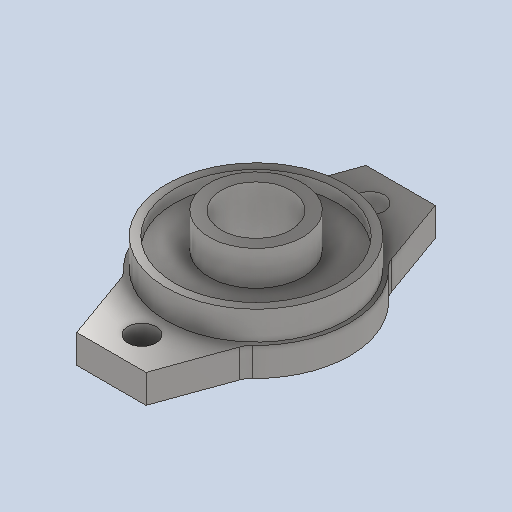
# Autodesk Inventor part: HCMUTE-CDT23-GOI_DO_PHI-17
Saved by Autodesk Inventor 2023 (Build 270158000, 158)
## iProperties
Created: 2023-11-19
Part Number: HCMUTE-CDT23-GOI_DO_PHI-17
Material: Stainless Steel
Document SubType Name: Modeling
Designer: havie
Mass: 171.361 g
Surface Area: 85.9405 cm^2
Volume: 21.4202 cm^3
Density: 8 g/cm^3
Appearance: Semi-Polished
Author: havie
Autodesk Inventor part; units mm, degrees
ref_plane "YZ Plane" through (0, 0, 0) normal (1, 0, 0) x (0, 1, 0)
ref_plane "XZ Plane" through (0, 0, 0) normal (0, 1, 0) x (-1, 0, 0)
ref_plane "XY Plane" through (0, 0, 0) normal (0, 0, 1) x (1, 0, 0)
sketch "Sketch1" plane through (0, 0, 0) normal (0, 1, 0) x (-1, 0, 0)
  circle A0 centre (0, 0) radius 23
  dimension "d0" = 46
  constraints: 1 centre point, 1 coincident
  measures "d0" diameter of A0
extrude "Extrusion1" add sketch "Sketch1" along normal blind 7
sketch "Sketch2" plane through (0, 7, 0) normal (0, 1, 0) x (1, 0, 0)
  line L0 (-8.5, -35.5) -> (8.5, -35.5)
  line L1 (-8.5, -35.5) -> (-15, -17.4356)
  circle A0 centre (0, 0) radius 23 projected
  line L2 (8.5, -35.5) -> (15, -17.4356)
  circle A1 centre (0, -28) radius 3.5
  point P0 (0, -35.5)
  dimension "d3" = 17
  dimension "d4" = 35.5
  dimension "d5" = 7
  dimension "d6" = 28
  dimension "d7" = 30
  constraints: 6 end point, 2 point on circle, 2 vertical alignment, 1 centre point, 1 horizontal, 1 horizontal alignment, 1 midpoint
  measures "d3" distance of L0.start L0.end
  measures "d4" distance from line of point (0, 0) L0
  measures "d5" diameter of A1
  measures "d6" distance of point (0, 0) A1.centre
  measures "d7" distance of L2.end L1.end
extrude "Extrusion2" add sketch "Sketch2" against normal blind 7 contours L1 A0 L2 L0
fillet "Fillet1" radius 5 2 edges at (15, 3.5, 17.4356) (-15, 3.5, 17.4356)
mirror "Mirror1" about plane through (0, 0, 0) normal (0, 0, 1) of "Extrusion2", "Fillet1"
sketch "Sketch3" plane through (0, 7, 0) normal (0, 1, 0) x (1, 0, 0)
  circle A0 centre (0, 0) radius 22
  dimension "d11" = 44
  constraints: 1 centre point, 1 coincident
  measures "d11" diameter of A0
extrude "Extrusion3" add sketch "Sketch3" along normal blind 7
sketch "Sketch4" plane through (0, 14, 0) normal (0, 1, 0) x (1, 0, 0)
  circle A0 centre (0, 0) radius 11.5
  dimension "d14" = 23
  constraints: 1 centre point, 1 coincident
  measures "d14" diameter of A0
extrude "Extrusion4" add sketch "Sketch4" along normal blind 5.5
sketch "Sketch5" plane through (0, 19.5, 0) normal (0, 1, 0) x (1, 0, 0)
  circle A0 centre (0, 0) radius 8.5
  dimension "d17" = 17
  constraints: 1 centre point, 1 coincident
  measures "d17" diameter of A0
extrude "Extrusion5" cut sketch "Sketch5" against normal through all
sketch "Sketch6" plane through (0, 14, 0) normal (0, 1, 0) x (1, 0, 0)
  circle A0 centre (0, 0) radius 20
  circle A1 centre (0, 0) radius 11.5 projected
  dimension "d20" = 40
  constraints: 1 centre point, 1 coincident
  measures "d20" diameter of A0
extrude "Extrusion6" cut sketch "Sketch6" against normal blind 3
body "Solid1"
